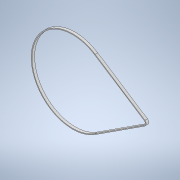
# Autodesk Inventor part: belt
Saved by Autodesk Inventor 2022 (Build 260153000, 153)
## iProperties
Created: 2022-01-31
Part Number: belt
Material: Generic
Document SubType Name: Modeling
Designer: Martijn
Density: 1 g/cm^3
Appearance: Default
Author: Martijn
Autodesk Inventor part; units mm, degrees
ref_plane "YZ Plane" through (0, 0, 0) normal (1, 0, 0) x (0, 1, 0)
ref_plane "XZ Plane" through (0, 0, 0) normal (0, 1, 0) x (-1, 0, 0)
ref_plane "XY Plane" through (0, 0, 0) normal (0, 0, 1) x (1, 0, 0)
sketch "Sketch1" plane through (0, 0, 0) normal (0, 0, 1) x (1, 0, 0)
  arc A0 (51.4063, 79.344) -> (51.4063, -79.344) centre (0, 0) ccw
  arc A1 (167.2707, -4.2764) -> (167.2707, 4.2764) centre (164.5, 0) ccw
  line L0 (51.4063, 79.344) -> (167.2707, 4.2764)
  line L1 (167.2707, -4.2764) -> (51.4063, -79.344)
  line L2 (-150.1688, 0) -> (225.2229, 0) projected
  arc A2 (52.4938, 81.0225) -> (52.4938, -81.0225) centre (0, 0) ccw
  arc A3 (168.3582, -5.9549) -> (168.3582, 5.9549) centre (164.5, 0) ccw
  line L3 (52.4938, 81.0225) -> (168.3582, 5.9549)
  line L4 (168.3582, -5.9549) -> (52.4938, -81.0225)
  dimension "d0" = 2
  dimension "d2" = 5.0955
  dimension "d5" = 94.5414
  dimension "d6" = 164.5
  constraints: 8 end point, 8 point on circle, 6 tangent, 4 centre point, 3 coincident, 2 parallel, 1 point on line
  measures "d0" distance between parallel lines of L0 L3
  measures "d2" radius of A1
  measures "d5" radius of A0
  measures "d6" distance of point (0, 0) A1.centre
extrude "Extrusion1" add sketch "Sketch1" along normal blind 6 contours A0 L2 A2 L3 A3 A1 L0 | A0 L1 A1 L2 A3 L4 A2
body "Solid1"
